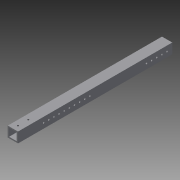
# Autodesk Inventor part: Clapper 15 in Segment (4)
Saved by Autodesk Inventor 2014 (Build 180170000, 170)
## iProperties
Created: 2014-02-24
Part Number: Clapper 15 in Segment (4)
Material: Generic
Document SubType Name: Sheet Metal
Designer: Michael
Density: 1 g/cm^3
Sheet Metal Rule: Default
Appearance: Default
Author: Michael
Autodesk Inventor part; units mm, degrees
ref_plane "YZ Plane" through (0, 0, 0) normal (1, 0, 0) x (0, 1, 0)
ref_plane "XZ Plane" through (0, 0, 0) normal (0, 1, 0) x (-1, 0, 0)
ref_plane "XY Plane" through (0, 0, 0) normal (0, 0, 1) x (1, 0, 0)
sketch "Sketch1" plane through (0, 0, 0) normal (0, 0, 1) x (1, 0, 0)
  line L0 (0, 0) -> (25.4, 0)
  line L1 (25.4, 0) -> (25.4, 25.4)
  line L2 (25.4, 25.4) -> (0, 25.4)
  line L3 (0, 25.4) -> (0, 0)
  line L4 (3.175, 22.225) -> (22.225, 22.225)
  line L5 (22.225, 22.225) -> (22.225, 3.175)
  line L6 (22.225, 3.175) -> (3.175, 3.175)
  line L7 (3.175, 3.175) -> (3.175, 22.225)
  dimension "d0" = 25.4
  dimension "d1" = 25.4
  dimension "d2" = 3.175
  constraints: 16 end point, 4 parallel, 2 perpendicular, 1 horizontal, 3 other
  measures "d0" distance of L2.end L1.end
  measures "d1" distance of L1.end L0.end
  measures "d2" distance between parallel lines of L2 L4
extrude "Extrusion1" add sketch "Sketch1" along normal blind 381
sketch "Sketch2" plane through (25.4, 0, 0) normal (1, 0, 0) x (0, 0, -1)
  line L0 (0, 0) -> (0, 25.4) projected
  line L1 (-381, 0) -> (-381, 25.4) projected
  line L2 (0, 0) -> (-381, 0) projected
  circle A0 centre (-317.5, 12.7) radius 2.0701
  circle A1 centre (-304.8, 12.7) radius 2.0701
  circle A2 centre (-292.1, 12.7) radius 2.0701
  circle A3 centre (-279.4, 12.7) radius 2.0701
  circle A4 centre (-266.7, 12.7) radius 2.0701
  circle A5 centre (-254, 12.7) radius 2.0701
  circle A6 centre (-241.3, 12.7) radius 2.0701
  circle A7 centre (-228.6, 12.7) radius 2.0701
  circle A8 centre (-215.9, 12.7) radius 2.0701
  circle A9 centre (-203.2, 12.7) radius 2.0701
  circle A10 centre (-12.7, 12.7) radius 2.0701
  circle A11 centre (-25.4, 12.7) radius 2.0701
  circle A12 centre (-38.1, 12.7) radius 2.0701
  circle A13 centre (-50.8, 12.7) radius 2.0701
  circle A14 centre (-63.5, 12.7) radius 2.0701
  dimension "d5" = 4.1402
  dimension "d6" = 12.7
  dimension "d7" = 63.5
  dimension "d10" = 12.7
  dimension "d15" = 12.7
  dimension "d16" = 12.7
  dimension "d19" = 12.7
  constraints: 15 centre point, 2 horizontal, 1 equal radius, 26 other
  measures "d5" diameter of A0
  measures "d6" distance from line of L2 A0.centre
  measures "d7" distance from line of L1 A0.centre
  measures "d10" distance of A0.centre A1.centre
  measures "d15" distance from line of L2 A10.centre
  measures "d16" distance from line of L0 A10.centre
  measures "d19" distance of A10.centre A11.centre
extrude "Extrusion2" cut sketch "Sketch2" against normal blind 381
sketch "Sketch3" plane through (0, 25.4, 0) normal (0, 1, 0) x (1, 0, 0)
  line L0 (0, 0) -> (0, -381) projected
  line L1 (25.4, -381) -> (0, -381) projected
  circle A0 centre (12.7, -368.3) radius 2.0701
  circle A1 centre (12.7, -342.9) radius 2.0701
  dimension "d26" = 4.1402
  dimension "d27" = 12.7
  dimension "d28" = 12.7
  dimension "d31" = 25.4
  constraints: 2 centre point, 1 vertical, 2 other
  measures "d26" diameter of A0
  measures "d27" distance from line of L0 A0.centre
  measures "d28" distance from line of L1 A0.centre
  measures "d31" distance of A0.centre A1.centre
extrude "Extrusion3" cut sketch "Sketch3" against normal blind 381
equation "\"BendRadius\" = Thickness"
equation "\"BendReliefWidth\" = Thickness"
equation "\"BendReliefDepth\" = 0.5 * Thickness"
equation "\"CornerReliefSize\" = 4 * Thickness"
equation "\"MinimumRemnant\" = 2 * Thickness"
equation "\"TransitionRadius\" = BendRadius"
equation "\"JacobiRadiusSize\" = BendRadius"
equation "\"GapSize\" = Thickness"
equation "\"Thickness\" = 3.048"
body "Solid1"
